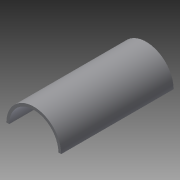
# Autodesk Inventor part: obudowa - klosz dla zarowki
Saved by Autodesk Inventor 2014 (Build 180170000, 170)
## iProperties
Created: 2018-02-27
Part Number: obudowa - klosz dla zarowki
Material: Generic
Document SubType Name: Modeling
Designer: HP820
Density: 1 g/cm^3
Appearance: Default
Author: HP820
Autodesk Inventor part; units mm, degrees
ref_plane "YZ Plane" through (0, 0, 0) normal (1, 0, 0) x (0, 1, 0)
ref_plane "XZ Plane" through (0, 0, 0) normal (0, 1, 0) x (-1, 0, 0)
ref_plane "XY Plane" through (0, 0, 0) normal (0, 0, 1) x (1, 0, 0)
sketch "Sketch1" plane through (0, 0, 0) normal (0, 1, 0) x (-1, 0, 0)
  arc A0 (35, 0) -> (-35, 0) centre (0, 0) ccw
  arc A1 (39, 0) -> (-39, 0) centre (0, 0) ccw
  line L0 (-39, 0) -> (-35, 0)
  line L1 (35, 0) -> (39, 0)
  dimension "d0" = 70
  dimension "d1" = 78
  constraints: 4 end point, 4 point on circle, 2 centre point, 2 coincident, 1 collinear
  measures "d0" diameter of A0
  measures "d1" diameter of A1
extrude "Extrusion1" add sketch "Sketch1" along normal blind 160
body "Solid1"
